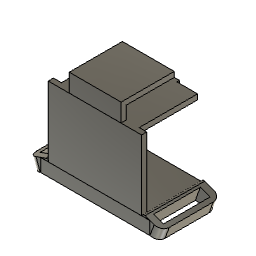
project_holder v5 (Autodesk Fusion 360 design; units mm, degrees)
Autodesk Fusion 360 part; units mm, degrees
sketch "Sketch1" plane through (0, 0, 0) normal (0, 0, 1) x (1, 0, 0)
  line L0 (-21, 11.5) -> (21, 11.5)
  line L1 (21, 11.5) -> (21, -11.5)
  line L2 (21, -11.5) -> (-21, -11.5)
  line L3 (-21, -11.5) -> (-21, 11.5)
  line L4 (-21, 11.5) -> (21, -11.5) construction
  line L5 (21, 11.5) -> (-21, -11.5) construction
  dimension "d1" = 42
  dimension "d2" = 23
  constraint horizontal L0
  constraint perpendicular L0 L1
  constraint parallel L0 L2
  constraint parallel L1 L3
  constraint coincident L4 origin
  constraint coincident L5 origin
  measures "d1" distance of L1.end L2.end
  measures "d2" distance of L0.end L1.end
extrude "Extrude1" add sketch "Sketch1" along normal blind 5
sketch "Sketch3" plane through (0, 0, 5) normal (0, 0, 1) x (-1, 0, 0)
  line L0 (21, 11.5) -> (-21, 11.5)
  line L1 (-21, 11.5) -> (-21, -11.5)
  line L2 (-21, -11.5) -> (21, -11.5)
  line L3 (21, -11.5) -> (21, 11.5)
  line L4 (-17.9148, 11.5098) -> (18.0852, 11.5098)
  line L5 (18.0852, 11.5098) -> (18.0852, 9.5098)
  line L6 (18.0852, 9.5098) -> (-17.9148, 9.5098)
  line L7 (-17.9148, 9.5098) -> (-17.9148, 11.5098)
  line L8 (-17.9148, 11.5098) -> (18.0852, 9.5098) construction
  line L9 (18.0852, 11.5098) -> (-17.9148, 9.5098) construction
  point P0 (0.0852, 10.5098)
  dimension "d44" = 36
  dimension "d45" = 2
  constraint horizontal L4
  constraint perpendicular L4 L5
  constraint parallel L4 L6
  constraint parallel L5 L7
  constraint coincident L8 P0
  constraint coincident L9 P0
  measures "d44" distance of L5.end L6.end
  measures "d45" distance of L4.end L5.end
extrude "Extrude3" add sketch "Sketch3" along normal blind 25 contours L0 L5 L6 L7 | L0 L4 L5 L7
sketch "Sketch4" plane through (0, 0, 30) normal (0, 0, 1) x (-1, 0, 0)
  line L0 (15, 10.5175) -> (-15, 10.5175)
  line L1 (-15, 10.5175) -> (-15, -13)
  line L2 (-15, -13) -> (15, -13)
  line L3 (15, -13) -> (15, 10.5175)
  line L4 (-17.9148, 9.5098) -> (18.0852, 9.5098)
  line L5 (18.0852, 9.5098) -> (18.0852, 11.5098)
  line L6 (18.0852, 11.5098) -> (-17.9148, 11.5098)
  line L7 (-17.9148, 11.5098) -> (-17.9148, 9.5098)
  constraint horizontal L0
  constraint vertical L1
  constraint horizontal L2
  constraint vertical L3
extrude "Extrude4" add sketch "Sketch4" along normal blind 2
ref_plane "WorkPlane1" through (21, 0, 5) normal (0.34202, 0, 0.939693) x (0, 1, 0)
sketch "Sketch7" plane through (4.0635, 0, 11.1644) normal (0.34202, 0, 0.939693) x (0, 1, 0)
  line L0 (-11.4455, -15.1007) -> (11.5394, -15.1007)
  line L1 (11.5394, -15.1007) -> (11.5394, -22.8179)
  line L2 (11.5394, -22.8179) -> (-11.4455, -22.8179)
  line L3 (-11.4455, -22.8179) -> (-11.4455, -15.1007)
  constraint horizontal L0
  constraint vertical L1
  constraint horizontal L2
  constraint vertical L3
extrude "Extrude7" add sketch "Sketch7" against normal blind 4.7
fillet "Fillet1" radius 3 2 edges at (24.7015, -11.4455, 1.1519) (24.7015, 11.5394, 1.1519)
fillet "Fillet2" radius 1 1 edges at (18.2536, 0.0469, 5.9996)
sketch "Sketch8" plane through (4.0635, 0, 11.1644) normal (0.34202, 0, 0.939693) x (0, 1, 0)
  line L0 (11.5394, -16.1007) -> (-11.4455, -16.1007)
  line L1 (-8.4455, -22.8179) -> (8.5394, -22.8179)
  arc A0 (8.5394, -22.8179) -> (11.5394, -19.8179) centre (8.5394, -19.8179) ccw
  line L2 (11.5394, -19.8179) -> (11.5394, -16.1007)
  line L3 (-9, -17.0226) -> (9, -17.0226)
  line L4 (9, -17.0226) -> (9, -21.0226)
  line L5 (9, -21.0226) -> (-9, -21.0226)
  line L6 (-9, -21.0226) -> (-9, -17.0226)
  line L7 (-11.4455, -16.1007) -> (-11.4455, -18.0234)
  line L8 (-11.4455, -18.0234) -> (-11.4455, -19.8179)
  arc A1 (-11.4455, -19.8179) -> (-8.4455, -22.8179) centre (-8.4455, -19.8179) ccw
  constraint horizontal L3
  constraint vertical L4
  constraint horizontal L5
  constraint vertical L6
extrude "Extrude8" cut sketch "Sketch8" against normal blind 8 contours L3 L4 L5 L6
ref_plane "WorkPlane2" through (-21, 0, 5) normal (-0.34202, 0, 0.939693) x (0, -1, 0)
sketch "Sketch9" plane through (4.0635, 0, 11.1644) normal (0.34202, 0, 0.939693) x (0, 1, 0)
sketch "Sketch10" plane through (-4.0635, 0, 11.1644) normal (-0.34202, 0, 0.939693) x (0, -1, 0)
  line L0 (11.4414, -15.0071) -> (-11.5436, -15.0071)
  line L1 (-11.5436, -15.0071) -> (-11.5436, -22.9991)
  line L2 (-11.5436, -22.9991) -> (11.4414, -22.9991)
  line L3 (11.4414, -22.9991) -> (11.4414, -15.0071)
  dimension "d29" = 22.985
  dimension "d30" = 7.992
  constraint horizontal L0
  constraint vertical L1
  constraint horizontal L2
  constraint vertical L3
  measures "d29" distance of L0.start L0.end
  measures "d30" distance of L0.start L2.end
extrude "Extrude9" add sketch "Sketch10" against normal blind 4.7
fillet "Fillet3" radius 3 2 edges at (-24.8718, -11.4414, 1.09) (-24.8718, 11.5436, 1.09)
sketch "Sketch11" plane through (4.0635, 0, 11.1644) normal (0.34202, 0, 0.939693) x (0, 1, 0)
sketch "Sketch12" plane through (-4.0635, 0, 11.1644) normal (-0.34202, 0, 0.939693) x (0, -1, 0)
  arc A0 (-11.5436, -19.9991) -> (-8.5436, -22.9991) centre (-8.5436, -19.9991) ccw
  line L0 (-8.5436, -22.9991) -> (8.4414, -22.9991)
  line L1 (11.4414, -19.9991) -> (11.4414, -18.0234)
  line L2 (11.4414, -15.0071) -> (-11.5436, -15.0071)
  line L3 (-11.5436, -15.0071) -> (-11.5436, -19.9991)
  line L4 (-9.1832, -17.1141) -> (8.8168, -17.1141)
  line L5 (8.8168, -17.1141) -> (8.8168, -21.1141)
  line L6 (8.8168, -21.1141) -> (-9.1832, -21.1141)
  line L7 (-9.1832, -21.1141) -> (-9.1832, -17.1141)
  arc A1 (8.4414, -22.9991) -> (11.4414, -19.9991) centre (8.4414, -19.9991) ccw
  line L8 (11.4414, -18.0234) -> (11.4414, -15.0071)
  dimension "d35" = 18
  dimension "d36" = 4
  constraint horizontal L4
  constraint vertical L5
  constraint horizontal L6
  constraint vertical L7
  measures "d35" distance of L4.start L4.end
  measures "d36" distance of L4.start L6.end
extrude "Extrude10" cut sketch "Sketch12" against normal blind 15 contours L4 L5 L6 L7
sketch "Sketch15" plane through (0, 13, 0) normal (0, 1, 0) x (-1, 0, 0)
  line L0 (-15, 30) -> (15, 30)
  line L1 (15, 30) -> (15, 32)
  line L2 (15, 32) -> (-15, 32)
  line L3 (-15, 32) -> (-15, 30)
  line L4 (-7, 32) -> (15, 32)
  line L5 (15, 32) -> (15, 23)
  line L6 (15, 23) -> (-7, 23)
  line L7 (-7, 23) -> (-7, 32)
  constraint horizontal L4
  constraint vertical L5
  constraint horizontal L6
  constraint vertical L7
  constraint coincident L2 L4.start
extrude "Extrude12" add sketch "Sketch15" along normal blind 1 contours L0 L1 L2 L4 L5 L7 | L0 L5 L6 L7
fillet "Fillet4" radius 1 1 edges at (-18.1656, 0.0511, 6.0317)
ref_plane "WorkPlane3" through (0, -11.5, 0) normal (0, 1, 0) x (0, 0, 1)
sketch "Sketch18" plane through (0, -11.5, 0) normal (0, 1, 0) x (1, 0, 0)
  line L0 (-10, -32) -> (10, -32)
  line L1 (10, -32) -> (10, -37)
  line L2 (10, -37) -> (-10, -37)
  line L3 (-10, -37) -> (-10, -32)
  constraint horizontal L0
  constraint vertical L1
  constraint horizontal L2
  constraint vertical L3
extrude "Extrude13" add sketch "Sketch18" along normal blind 2
sketch "Sketch19" plane through (0, 0, 37) normal (0, 0, 1) x (-1, 0, 0)
  line L0 (10, 11.5) -> (-10, 11.5)
  line L1 (-10, 11.5) -> (-10, 9.5)
  line L2 (-10, 9.5) -> (10, 9.5)
  line L3 (10, 9.5) -> (10, 11.5)
  line L4 (10, 11.5) -> (-10, 11.5)
  line L5 (-10, 11.5) -> (-10, -9)
  line L6 (-10, -9) -> (10, -9)
  line L7 (10, -9) -> (10, 11.5)
  constraint horizontal L4
  constraint vertical L5
  constraint horizontal L6
  constraint vertical L7
  constraint coincident L0.start L3.end
extrude "Extrude14" add sketch "Sketch19" along normal blind 2
